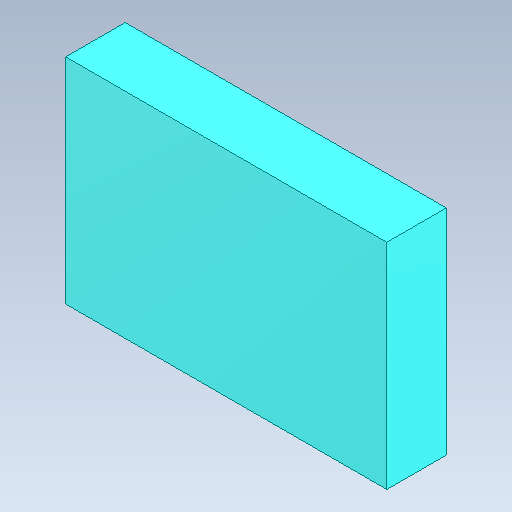
# Autodesk Inventor part: NX5032GA
Saved by Autodesk Inventor 2021 (Build 250183000, 183)
## iProperties
Created: 2020-11-03
Part Number: NX5032GA
Material: Generic
Document SubType Name: Modeling
Designer: faiya
Density: 1 g/cm^3
Appearance: 2-SMD-5X3, NX5032GA
Author: faiya
Autodesk Inventor part; units mm, degrees
ref_plane "YZ Plane" through (0, 0, 0) normal (1, 0, 0) x (0, 1, 0)
ref_plane "XZ Plane" through (0, 0, 0) normal (0, 1, 0) x (-1, 0, 0)
ref_plane "XY Plane" through (0, 0, 0) normal (0, 0, 1) x (1, 0, 0)
sketch "2-SMD-5X3, NX5032GA_37" plane through (0, 0, 0) normal (0, 0, 1) x (1, 0, 0)
  line L0 (-2.7, 1.8) -> (2.7, 1.8)
  line L1 (2.7, 1.8) -> (2.7, -1.8)
  line L2 (2.7, -1.8) -> (-2.7, -1.8)
  line L3 (-2.7, -1.8) -> (-2.7, 1.8)
  constraints: 8 end point
extrude "Extrusion1" add sketch "2-SMD-5X3, NX5032GA_37" along normal blind 1
body "Solid1"
